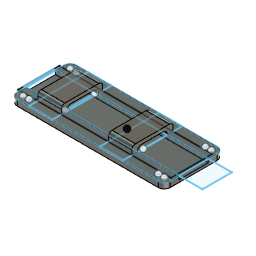
LoquetVerrou (Autodesk Fusion 360 archive; units mm, degrees)
design "VerrouPart2"
Autodesk Fusion 360 part; units mm, degrees
sketch "Esquisse1" plane through (0, 0, 0) normal (0, 0, 1) x (1, 0, 0)
  line L0 (51.6129, 25) -> (-68.3871, 25)
  line L1 (-73.3871, 20) -> (-73.3871, -20)
  line L2 (-68.3871, -25) -> (51.6129, -25)
  line L3 (56.6129, -20) -> (56.6129, 20)
  line L4 (-58.3871, 25) -> (-38.3871, 25)
  line L5 (-38.3871, 25) -> (-38.3871, -25)
  line L6 (-38.3871, -25) -> (-58.3871, -25)
  line L7 (-58.3871, -25) -> (-58.3871, 25)
  line L8 (1.6129, 25) -> (21.6129, 25)
  line L9 (21.6129, 25) -> (21.6129, -25)
  line L10 (21.6129, -25) -> (1.6129, -25)
  line L11 (1.6129, -25) -> (1.6129, 25)
  line L12 (55, -17.5) -> (-75, -17.5)
  line L13 (-75, -17.5) -> (-75, 17.5)
  line L14 (-75, 17.5) -> (55, 17.5)
  line L15 (55, 17.5) -> (55, -17.5)
  line L16 (-40, -12.5) -> (-40, 12.5)
  line L17 (21.6129, 7.8125) -> (21.6129, -7.8125)
  arc A0 (-68.3871, 25) -> (-73.3871, 20) centre (-68.3871, 20) ccw
  arc A1 (56.6129, 20) -> (51.6129, 25) centre (51.6129, 20) ccw
  arc A2 (51.6129, -25) -> (56.6129, -20) centre (51.6129, -20) ccw
  arc A3 (-73.3871, -20) -> (-68.3871, -25) centre (-68.3871, -20) ccw
  line L18 (76.6129, -12.5) -> (-75, -12.5)
  line L19 (-75, -12.5) -> (-75, 12.5)
  line L20 (-75, 12.5) -> (76.6129, 12.5)
  line L21 (76.6129, 12.5) -> (76.6129, -12.5)
  circle A4 centre (46.6129, 20) radius 2.5
  circle A5 centre (46.6129, -20) radius 2.5
  circle A6 centre (-63.3871, 20) radius 2.5
  circle A7 centre (-63.3871, -20) radius 2.5
  dimension "d3" = 20
  dimension "d4" = 15
  dimension "d5" = 20
  dimension "d6" = 50
  dimension "d8" = 35
  dimension "d9" = 25
  dimension "d16" = 5
  dimension "d17" = 5
  dimension "d18" = 5
  dimension "d19" = 5
  dimension "d50" = 40
  dimension "d55" = 130
  dimension "d99" = 25
  dimension "d106" = 150
  dimension "d107" = 130
  dimension "d115" = 5
  dimension "d116" = 10
  dimension "d117" = 5
  dimension "d118" = 10
  dimension "d119" = 5
  dimension "d120" = 5
  dimension "d121" = 10
  dimension "d122" = 10
  constraint horizontal L0
  constraint perpendicular L0 L1
  constraint parallel L0 L2
  constraint parallel L1 L3
  constraint horizontal L4
  constraint vertical L5
  constraint horizontal L6
  constraint vertical L7
  constraint coincident L0 L4.start
  constraint horizontal L8
  constraint vertical L9
  constraint horizontal L10
  constraint vertical L11
  constraint coincident L0 L8.start
  constraint horizontal L12
  constraint perpendicular L12 L13
  constraint parallel L12 L14
  constraint parallel L13 L15
  constraint tangent L0 A0
  constraint tangent L1 A0
  constraint tangent L0 A1
  constraint tangent L3 A1
  constraint tangent L3 A2
  constraint tangent L2 A2
  constraint tangent L1 A3
  constraint tangent L2 A3
  constraint coincident L9 L17.start
  constraint horizontal L18
  constraint perpendicular L18 L19
  constraint parallel L18 L20
  constraint parallel L19 L21
  measures "d3" distance of L4.start L4.end
  measures "d4" distance of L1 L7
  measures "d5" distance of L8.start L8.end
  measures "d6" distance of L8.start L10.end
  measures "d8" distance of L12.end L13.end
  measures "d9" distance of L16.start L16.end
  measures "d16" radius of A0
  measures "d17" radius of A1
  measures "d18" radius of A2
  measures "d19" radius of A3
  measures "d50" distance of L5 L11
  measures "d55" distance of L12.start L12.end
  measures "d99" distance of L18.end L19.end
  measures "d106" distance of L1 L21
  measures "d107" distance of L1.start L3.end
  measures "d115" diameter of A4
  measures "d116" distance of L3.end A4.centre
  measures "d117" diameter of A5
  measures "d118" distance of L3.start A5.centre
  measures "d119" diameter of A6
  measures "d120" diameter of A7
  measures "d121" distance of L1.start A6.centre
  measures "d122" distance of L1.end A7.centre
extrude "Extrusion14" add sketch "Esquisse1" against normal blind 5 contours A4 | L0 L3 L9 L14 L15 A1 L20 | L0 L8 L9 L11 L14 | L0 L5 L11 L14 | L9 L14 L15 L20 | L9 L11 L14 L20 | L3 L15 L18 L20 | L0 L4 L5 L7 L14 | L5 L11 L14 L20 | L9 L15 L17 L18 L20 | L9 L11 L17 L18 L20 | A5 | L2 L3 L9 L12 L15 A2 L18 | A6 | L0 L1 L7 L14 A0 | L5 L7 L14 L20 | L5 L11 L18 L20 | L9 L12 L15 L18 | L1 L7 L14 L20 | L5 L16 L18 L20 | L9 L11 L12 L18 | L5 L11 L12 L18 | L7 L16 L18 L20 | L1 L7 L18 L20 | L5 L7 L12 L18 | L2 L9 L10 L11 L12 | L2 L5 L11 L12 | L1 L7 L12 L18 | L2 L5 L6 L7 L12 | A7 | L1 L2 L7 L12 A3
extrude "Extrusion15" cut sketch "Esquisse1" against normal blind 3 contours L5 L11 L14 L20 | L9 L11 L17 L18 L20 | L5 L16 L18 L20
extrude "Extrusion16" cut 1 faces at (-40, -4.1667, -1) along direction (-1, 0, 0) blind 20
extrude "Extrusion17" cut 1 faces at (21.6129, 4.1667, -1) along direction (1, 0, 0) blind 20
extrude "Extrusion18" add sketch "Esquisse1" along normal blind 7 contours L9 L11 L14 L20 | L9 L11 L17 L18 L20 | L5 L7 L14 L20 | L5 L16 L18 L20 | L9 L11 L12 L18 | L7 L16 L18 L20 | L5 L7 L12 L18
extrude "Extrusion19" cut 1 faces at (8.2796, -4.1667, 0) along direction (0, 0, 1) blind 4
extrude "Extrusion20" cut 1 faces at (-45.0538, 4.1667, 0) along direction (0, 0, 1) blind 4
fillet "Congé6" radius 3 4 edges at (-48.3871, -17.5, 7) (-48.3871, 17.5, 7) (11.6129, -17.5, 7) (11.6129, 17.5, 7)
hole "Perçage5" at (46.6129, -20, 0) at (46.6129, 20, 0) at (-63.3871, -20, 0) at (-63.3871, 20, 0) direction (0, 0, -1) diameter 5 depth 5 tip angle 180 counterbore diameter 5.5 counterbore depth 2
extrude "Extrusion21" cut 1 faces at (41.6129, 4.1667, -1) along direction (1, 0, 0) blind 15
extrude "Extrusion22" cut 1 faces at (-60, -4.1667, -1) along direction (-1, 0, 0) blind 15
extrude "Extrusion25" add 1 faces at (-25.0538, 15.8333, -3) along direction (0, 0, 1) blind 3
extrude "Extrusion26" cut 1 faces at (-38.3871, 4.1667, -2) along direction (1, 0, 0) blind 95
fillet "Congé10" radius 3 2 edges at (11.6129, 12.5, 4) (-48.3871, 12.5, 4)
fillet "Congé11" radius 3 2 edges at (-48.3871, -12.5, 4) (11.6129, -12.5, 4)

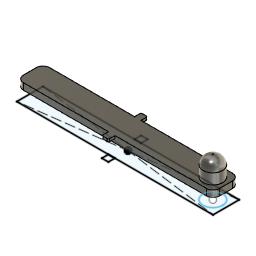
design "VerrouPart3"
Autodesk Fusion 360 part; units mm, degrees
sketch "Esquisse1" plane through (0, 0, 0) normal (0, 0, 1) x (1, 0, 0)
  line L0 (75, 10) -> (-75, 10)
  line L1 (-75, 10) -> (-75, -10)
  line L2 (-75, -10) -> (75, -10)
  line L3 (75, -10) -> (75, 10)
  line L4 (75, 10) -> (-75, -10) construction
  line L5 (-75, 10) -> (75, -10) construction
  line L6 (-5, 10) -> (0, 10)
  line L7 (0, 10) -> (0, 15)
  line L8 (0, 15) -> (-5, 15)
  line L9 (-5, 15) -> (-5, 10)
  line L10 (-5, -10) -> (0, -10)
  line L11 (0, -10) -> (0, -15)
  line L12 (0, -15) -> (-5, -15)
  line L13 (-5, -15) -> (-5, -10)
  circle A0 centre (64.8598, 0) radius 7.5
  dimension "d1" = 150
  dimension "d2" = 20
  dimension "d3" = 5
  dimension "d4" = 5
  dimension "d5" = 70
  dimension "d6" = 5
  dimension "d7" = 5
  dimension "d8" = 15
  dimension "d35" = 70
  constraint horizontal L0
  constraint perpendicular L0 L1
  constraint parallel L0 L2
  constraint parallel L1 L3
  constraint coincident L4 origin
  constraint coincident L5 origin
  constraint horizontal L6
  constraint vertical L7
  constraint horizontal L8
  constraint vertical L9
  constraint coincident L0 L6.start
  constraint horizontal L10
  constraint vertical L11
  constraint horizontal L12
  constraint vertical L13
  constraint coincident L2 L10.start
  measures "d1" distance of L1.end L2.end
  measures "d2" distance of L0.end L1.end
  measures "d3" distance of L6.start L6.end
  measures "d4" distance of L6.start L8.end
  measures "d5" distance of L0.end L9
  measures "d6" distance of L10.start L10.end
  measures "d7" distance of L10.start L12.end
  measures "d8" diameter of A0
  measures "d35" distance of L1 L13
extrude "Extrusion1" add sketch "Esquisse1" along normal blind 15
extrude "Extrusion2" cut sketch "Esquisse1" along normal blind 6 contours L0 L6 L7 L8 L9 | L2 L10 L11 L12 L13
fillet "Congé1" radius 5 4 edges at (-75, 10, 7.5) (-75, -10, 7.5) (75, 10, 7.5) (75, -10, 7.5)
extrude "Extrusion3" cut sketch "Esquisse1" along normal blind 3 contours L0 L1 L2 L3 L6 L10
extrude "Extrusion4" cut 2 faces at (-3.3333, -11.6667, 6) (-1.6667, 11.6667, 6) along direction (0, 0, 1) blind 4
fillet "Congé2" radius 1 4 edges at (-5, -15, 12.5) (0, -15, 12.5) (-5, 15, 12.5) (0, 15, 12.5)
extrude "Extrusion5" add sketch "Esquisse1" along normal blind 30 contours A0
extrude "Extrusion6" cut sketch "Esquisse1" along normal blind 3 contours A0
fillet "Congé3" radius 7 1 edges at (57.8673, -2.7121, 30)
extrude "Extrusion7" cut 1 faces at (23.3333, -3.3333, 3) along direction (0, 0, 1) blind 5
extrude "Extrusion8" cut 1 faces at (23.3333, -3.3333, 8) along direction (0, 0, 1) blind 1
extrude "Extrusion9" cut 2 faces at (-3.3333, -11.3333, 10) (-3.3333, 11.3333, 10) along direction (0, 0, 1) blind 3
extrude "Extrusion10" cut 1 faces at (23.3333, -3.3333, 9) along direction (0, 0, 1) blind 1
